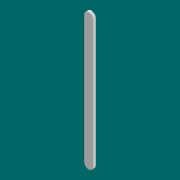
# Autodesk Inventor part: stab
Saved by Autodesk Inventor 2020.1 (Build 241239000, 239)
## iProperties
Created: 2020-01-27
Part Number: stab
Material: Generic
Document SubType Name: Modeling
Designer: Pluscrafter
Density: 1 g/cm^3
Appearance: Default
Author: Pluscrafter
Autodesk Inventor part; units mm, degrees
ref_plane "YZ Plane" through (0, 0, 0) normal (1, 0, 0) x (0, 1, 0)
ref_plane "XZ Plane" through (0, 0, 0) normal (0, 1, 0) x (-1, 0, 0)
ref_plane "XY Plane" through (0, 0, 0) normal (0, 0, 1) x (1, 0, 0)
sketch "Sketch1" plane through (0, 0, 0) normal (0, 0, 1) x (1, 0, 0)
  line L0 (9.8, 4.9) -> (9.8, 145.1)
  line L1 (0, 145.1) -> (0, 4.9)
  line L2 (4.9, 150) -> (4.9, 0) construction
  arc A0 (9.8, 145.1) -> (0, 145.1) centre (4.9, 145.1) ccw
  arc A1 (0, 4.9) -> (9.8, 4.9) centre (4.9, 4.9) ccw
  point P0 (0, 0)
  dimension "d0" = 9.8
  constraints: 6 end point, 6 point on circle, 2 centre point, 2 coincident, 2 point on line, 1 parallel
  measures "d0" distance between parallel lines of L0 L1
extrude "Extrusion1" add sketch "Sketch1" along normal blind 3
body "Solid1"
